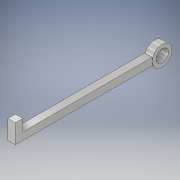
# Autodesk Inventor part: LegCathode
Saved by Autodesk Inventor 2019.3 (Build 233278000, 278)
## iProperties
Created: 2019-01-06
Part Number: LegCathode
Material: Aluminium 6061
Document SubType Name: Modeling
Designer: Jonas
Density: 2.7 g/cm^3
Appearance: Aluminium - poliert
Author: Jonas
Autodesk Inventor part; units mm, degrees
ref_plane "YZ Plane" through (0, 0, 0) normal (1, 0, 0) x (0, 1, 0)
ref_plane "XZ Plane" through (0, 0, 0) normal (0, 1, 0) x (-1, 0, 0)
ref_plane "XY Plane" through (0, 0, 0) normal (0, 0, 1) x (1, 0, 0)
sketch "Skizze1" plane through (0, 0, 0) normal (1, 0, 0) x (0, 1, 0)
  line L0 (1.7833, -0.9542) -> (0.85, -0.9542)
  line L1 (0.85, -0.9542) -> (0.85, -11.3542)
  line L2 (0.85, -11.3542) -> (0.25, -11.3542)
  line L3 (0.25, -11.3542) -> (0.25, -0.3542)
  line L4 (0.25, -0.3542) -> (1.7833, -0.3542)
  line L5 (1.7833, -0.3542) -> (1.7833, -0.9542)
  circle A0 centre (0.55, -12.1542) radius 0.8
  point P0 (0, 0)
  dimension "d0" = 0.6
  dimension "d1" = 0.6
  dimension "d2" = 11
  dimension "d8" = 1.6
  constraints: 12 end point, 5 perpendicular, 1 centre point, 1 horizontal, 1 tangent
  measures "d0" distance between parallel lines of L3 L1
  measures "d1" distance between parallel lines of L0 L4
  measures "d2" distance between parallel lines of L2 L4
  measures "d8" diameter of A0
extrude "Extrusion1" add sketch "Skizze1" along normal blind 0.6
sketch "Skizze4" plane through (0.6, 0.55, -12.1542) normal (1, 0, 0) x (0, 0, -1)
  circle A0 centre (0, 0) radius 0.5
  circle A1 centre (0, 0) radius 0.8 projected
  point P0 (-12.1542, -0.55)
  point P1 (-0.8, 0)
  dimension "d10" = 1
  constraints: 1 centre point, 1 horizontal alignment, 1 other
  measures "d10" diameter of A0
extrude "Extrusion3" cut sketch "Skizze4" against normal blind 0.6 contours A0
